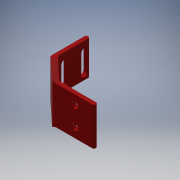
# Autodesk Inventor part: Y-Endstop holder
Saved by Autodesk Inventor 2018 (Build 220112000, 112)
## iProperties
Created: 2017-10-08
Part Number: Y-Endstop holder
Material: ABS-Kunststoff
Document SubType Name: Modeling
Designer: Till
Density: 1.06 g/cm^3
Appearance: Rot
Author: Till
Autodesk Inventor part; units mm, degrees
ref_plane "YZ Plane" through (0, 0, 0) normal (1, 0, 0) x (0, 1, 0)
ref_plane "XZ Plane" through (0, 0, 0) normal (0, 1, 0) x (-1, 0, 0)
ref_plane "XY Plane" through (0, 0, 0) normal (0, 0, 1) x (1, 0, 0)
sketch "Skizze1" plane through (0, 0, 0) normal (0, 0, 1) x (1, 0, 0)
  line L0 (0, 0) -> (20, 0)
  line L1 (20, 0) -> (20, 2)
  line L2 (20, 2) -> (0, 2)
  line L3 (0, 2) -> (-24, 25)
  line L4 (-24, 25) -> (-24, 42)
  line L5 (-24, 42) -> (-26, 42)
  line L6 (-26, 42) -> (-26, 23)
  line L7 (-26, 23) -> (-2, 0)
  line L8 (-2, 0) -> (0, 0)
  dimension "d0" = 20
  dimension "d1" = 2
  dimension "d2" = 17
  dimension "d3" = 2
  dimension "d4" = 90
  dimension "d5" = 19
  dimension "d6" = 90
  dimension "d9" = 26
  dimension "d10" = 0
  dimension "d11" = 42
  constraints: 18 end point, 3 parallel, 3 perpendicular, 1 collinear, 1 horizontal, 1 point on line
  measures "d0" distance of L0.start L0.end
  measures "d1" distance of L0.end L1.end
  measures "d2" distance of L3.end L4.end
  measures "d3" distance of L4.end L5.end
  measures "d4" angle of L5 L4
  measures "d5" distance of L5.end L6.end
  measures "d6" angle of L6 L5
  measures "d9" distance from line of L2.end L6
  measures "d10" horizontal distance of L0.start L2.end
  measures "d11" distance from line of L0.start L5
extrude "Extrusion1" add sketch "Skizze1" along normal blind 30
sketch "Skizze2" plane through (0, 2, 0) normal (0, 1, 0) x (1, 0, 0)
  circle A0 centre (10, -15) radius 1.6
  circle A1 centre (10, -25) radius 1.6
  line L0 (20, -30) -> (0, -30) projected
  line L1 (20, 0) -> (0, 0) projected
  line L2 (20, 0) -> (20, -30) projected
  dimension "d12" = 3.2
  dimension "d13" = 3.2
  dimension "d14" = 5
  dimension "d16" = 10
  dimension "d17" = 10
  dimension "d20" = 10
  constraints: 2 centre point
  measures "d12" diameter of A0
  measures "d13" diameter of A1
  measures "d14" distance from line of L0 A1.centre
  measures "d16" distance from line of L2 A0.centre
  measures "d17" distance from line of L2 A1.centre
  measures "d20" distance of A1.centre A0.centre
extrude "Extrusion2" cut sketch "Skizze2" against normal through all
sketch "Skizze5" plane through (-26, 42, 0) normal (0, 1, 0) x (1, 0, 0)
  line L0 (46.7536, 0) -> (46.7536, -10)
  line L1 (46.7536, -10) -> (26, -10)
  line L2 (26, 0) -> (26, -30) projected
  line L3 (46.7536, 0) -> (2, 0)
  line L4 (2, 0) -> (26, -10)
  point P0 (0, 0)
  dimension "d32" = 10
  dimension "d34" = 2
  constraints: 8 end point, 1 horizontal, 1 perpendicular, 1 point on line
  measures "d32" distance of L0.start L0.end
  measures "d34" distance of point (0, 0) L3.end
extrude "Extrusion5" cut sketch "Skizze5" against normal through all
sketch "Skizze6" plane through (-24, 25, 30) normal (1, 0, 0) x (0, 0, -1)
  line L0 (27, 3.5) -> (17, 3.5) construction
  line L1 (27, 5.1) -> (17, 5.1)
  line L2 (17, 1.9) -> (27, 1.9)
  arc A0 (27, 1.9) -> (27, 5.1) centre (27, 3.5) ccw
  arc A1 (17, 5.1) -> (17, 1.9) centre (17, 3.5) ccw
  line L3 (30, 0) -> (30, 17) projected
  line L4 (27, 14) -> (17, 14) construction
  line L5 (27, 15.6) -> (17, 15.6)
  line L6 (17, 12.4) -> (27, 12.4)
  arc A2 (27, 12.4) -> (27, 15.6) centre (27, 14) ccw
  arc A3 (17, 15.6) -> (17, 12.4) centre (17, 14) ccw
  line L7 (30, 17) -> (0, 17) projected
  line L8 (0, 0) -> (0, 17) projected
  point P0 (30, -25)
  point P1 (22, 3.5)
  point P2 (22, 14)
  dimension "d38" = 3.2
  dimension "d39" = 10
  dimension "d41" = 3.2
  dimension "d42" = 10.5
  dimension "d43" = 3
  dimension "d48" = 17
  constraints: 16 end point, 8 point on circle, 8 tangent, 4 centre point, 2 horizontal, 2 midpoint, 2 parallel
  measures "d38" diameter of A1
  measures "d39" distance of L0.start L0.end
  measures "d41" diameter of A3
  measures "d42" distance of point (22, 3.5) point (22, 14)
  measures "d43" distance from line of L7 point (22, 14)
  measures "d48" distance from line of L8 L0.end
extrude "Extrusion6" cut sketch "Skizze6" against normal through all
sketch "Skizze9" plane through (-26, 23, 0) normal (-1, 0, 0) x (0, 0, 1)
  line L0 (0, 19) -> (30, 19) projected
  line L1 (30, 19) -> (18, 19)
  line L2 (18, 19) -> (18, 0)
  line L3 (0, 0) -> (30, 0) projected
  line L4 (30, 19) -> (30, -23)
  line L5 (30, 0) -> (30, -23) projected
  line L6 (9.1667, -23) -> (30, -23) projected
  line L7 (23.4, -21) -> (26.6, -21) projected
  line L8 (30, -23) -> (18, 0)
  point P0 (0, -23)
  dimension "d54" = 12
  dimension "d55" = 0
  dimension "d56" = 0
  constraints: 8 end point, 3 point on line, 1 horizontal, 1 perpendicular, 3 other
  measures "d54" distance of L0.end L1.end
  measures "d55" distance from line of L6 L4.end
  measures "d56" distance of L4.end L8.start
extrude "Extrusion8" cut sketch "Skizze9" against normal up to surface (26 mm away)
fillet "Rundung3" radius 2 4 edges at (-24, 25, 9) (0, 2, 19.4783) (-26, 23, 9) (-2, 0, 19.5833)
fillet "Rundung3" radius 0.8 4 edges at (20, 0, 20) (20, 2, 20) (-24, 42, 9) (-26, 42, 9)
